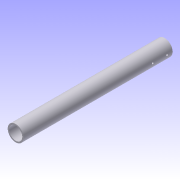
# Autodesk Inventor part: FE-00006-05
Saved by Autodesk Inventor 2012 (Build 160160000, 160)
## iProperties
Created: 2008-05-25
Part Number: FE-00006-05
Document SubType Name: Modeling
Designer: firstuser
Density: 1 g/cm^3
Mass: 169.448 g
Surface Area: 961.746 cm^2
Volume: 169.448 cm^3
Material: Default
Author: firstuser
Autodesk Inventor part; units mm, degrees
ref_plane "XZ Plane" through (0, 0, 0) normal (0, 1, 0) x (-1, 0, 0)
ref_plane "XY Plane" through (0, 0, 0) normal (0, 0, 1) x (1, 0, 0)
sketch "Sketch1" plane through (0, 0, 0) normal (0, 0, 1) x (1, 0, 0)
  circle A0 centre (0, 0) radius 21.0312
  circle A1 centre (0, 0) radius 17.4625
  dimension "d0" = 34.925
  dimension "d1" = 42.0624
  constraints: 2 centre point, 1 coincident
  measures "d0" diameter of A1
  measures "d1" diameter of A0
extrude "Extrusion1" add sketch "Sketch1" along normal blind 393.7
ref_plane "Work Plane1" through (0, 0, 0) normal (1, 0, 0) x (0, 0, 1)
sketch "Sketch2" plane through (0, 0, 0) normal (1, 0, 0) x (0, 0, 1)
  line L0 (-78.74, 0) -> (472.44, 0) projected
  line L1 (0, -21.0312) -> (393.7, -21.0312) projected
  line L2 (0, 21.0312) -> (393.7, 21.0312) projected
  line L3 (0, -17.4625) -> (0, 17.4625) projected
  line L4 (0, 21.0312) -> (0, -21.0312) projected
  circle A0 centre (14.2875, 0) radius 2.3813
  circle A1 centre (52.3875, 0) radius 2.3813
  line L5 (393.7, 21.0312) -> (393.7, -21.0312) projected
  circle A2 centre (311.15, 0) radius 3.175
  circle A3 centre (361.95, 0) radius 3.175
  dimension "d5" = 14.2875
  dimension "d6" = 38.1
  dimension "d7" = 4.7625
  dimension "d10" = 6.35
  dimension "d11" = 6.35
  dimension "d12" = 50.8
  dimension "d13" = 31.75
  constraints: 4 centre point, 4 point on line, 1 equal radius
  measures "d5" distance from line of A0.centre L3
  measures "d6" distance of A1.centre A0.centre
  measures "d7" diameter of A1
  measures "d10" diameter of A3
  measures "d11" diameter of A2
  measures "d12" distance of A2.centre A3.centre
  measures "d13" distance from line of A3.centre L5
extrude "Extrusion2" cut sketch "Sketch2" against normal mid plane 393.7 contours A0 L0 | L0 A0 | A1 L0 | L0 A1
extrude "Extrusion3" cut sketch "Sketch2" against normal through all contours A2 L0 | L0 A2 | A3 L0 | L0 A3
body "Solid1"
